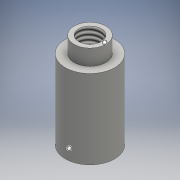
# Autodesk Inventor part: Standoff 7mm M2 Wurth 9774070243R
Saved by Autodesk Inventor 2016 (Build 200138000, 138)
## iProperties
Created: 2015-10-26
Part Number: Standoff 7mm M2 Wurth 9774070243R
Material: Generic
Document SubType Name: Modeling
Designer: jeremyhale
Density: 1 g/cm^3
Appearance: Default
Author: jeremyhale
Autodesk Inventor part; units mm, degrees
ref_plane "YZ Plane" through (0, 0, 0) normal (1, 0, 0) x (0, 1, 0)
ref_plane "XZ Plane" through (0, 0, 0) normal (0, 1, 0) x (-1, 0, 0)
ref_plane "XY Plane" through (0, 0, 0) normal (0, 0, 1) x (1, 0, 0)
sketch "Sketch1" plane through (0, 0, 0) normal (0, 1, 0) x (-1, 0, 0)
  line L0 (0, 0) -> (0, 8.4)
  line L1 (0, 8.4) -> (1.4, 8.4)
  line L2 (1.4, 8.4) -> (1.4, 7)
  line L3 (1.4, 7) -> (2.175, 7)
  line L4 (2.175, 7) -> (2.175, 0)
  line L5 (2.175, 0) -> (0, 0)
  line L6 (0, -1.68) -> (0, 10.08) projected
  dimension "d0" = 2.175
  dimension "d1" = 7
  dimension "d2" = 1.4
  dimension "d3" = 1.4
  constraints: 12 end point, 5 perpendicular, 1 vertical
  measures "d0" distance of L4.end L0.start
  measures "d1" distance of L3.end L4.end
  measures "d2" distance of L1.end L2.end
  measures "d3" distance of L0.end L1.end
revolve "Revolution1" add sketch "Sketch1" angle 360 about axis through (0, 0, -10) along (0, 0, 1)
hole "Hole1" at (0, 0, 8.4) direction (0, 0, -1) diameter 2 end through all
thread "Thread1" size "M2x0.4" class "6H" standard "ANSI Metric M Profile" full length
body "Solid1"
